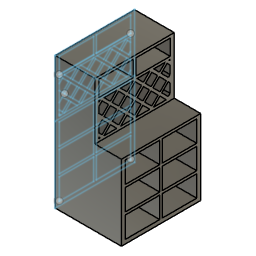
3D Plancha 7 (Autodesk Fusion 360 design; units mm, degrees)
Autodesk Fusion 360 part; units mm, degrees
sketch "Boceto1" plane through (0, 0, 0) normal (1, 0, 0) x (0, 1, 0)
  line L0 (47.0014, 109.9967) -> (107.0014, 109.9967)
  line L1 (107.0014, 109.9967) -> (107.0014, 9.9967)
  line L2 (107.0014, 9.9967) -> (47.0014, 9.9967)
  line L3 (47.0014, 9.9967) -> (47.0014, 109.9967)
  line L4 (47.0014, 66.9967) -> (107.0014, 66.9967)
  line L5 (104.0014, 13.7115) -> (104.0014, 13.2245)
  line L6 (50.0014, 13.2245) -> (50.0014, 13.7115)
  line L7 (76.0014, 64.9967) -> (76.0014, 48.9967)
  line L8 (78.0014, 64.9967) -> (78.0014, 48.9967)
  line L9 (50.0014, 48.9967) -> (76.0014, 48.9967)
  line L10 (78.0014, 48.9967) -> (104.0014, 48.9967)
  line L11 (50.0014, 64.9967) -> (76.0014, 64.9967)
  line L12 (78.0014, 64.9967) -> (104.0014, 64.9967)
  line L13 (76.0014, 46.9967) -> (76.0014, 30.9967)
  line L14 (78.0014, 46.9967) -> (78.0014, 30.9967)
  line L15 (76.0014, 28.9967) -> (76.0014, 12.9967)
  line L16 (78.0014, 28.9967) -> (78.0014, 12.9967)
  line L17 (50.0014, 30.9967) -> (76.0014, 30.9967)
  line L18 (78.0014, 30.9967) -> (104.0014, 30.9967)
  line L19 (50.0014, 12.9967) -> (76.0014, 12.9967)
  line L20 (78.0014, 12.9967) -> (104.0014, 12.9967)
  line L21 (50.0014, 46.9967) -> (76.0014, 46.9967)
  line L22 (78.0014, 46.9967) -> (104.0014, 46.9967)
  line L23 (104.0014, 64.9967) -> (104.0014, 48.9967)
  line L24 (50.0014, 28.9967) -> (76.0014, 28.9967)
  line L25 (78.0014, 28.9967) -> (104.0014, 28.9967)
  line L26 (104.0014, 46.9967) -> (104.0014, 30.9967)
  line L27 (104.0014, 28.9967) -> (104.0014, 12.9967)
  line L28 (50.0014, 12.9967) -> (50.0014, 28.9967)
  line L29 (50.0014, 30.9967) -> (50.0014, 46.9967)
  line L30 (50.0014, 48.9967) -> (50.0014, 64.9967)
  line L31 (103.8321, 93.9967) -> (103.8321, 68.9967)
  line L32 (103.8321, 68.9967) -> (50.0014, 68.9967)
  line L33 (50.0014, 68.9967) -> (50.0014, 93.9967)
  line L34 (104.0014, 107.9967) -> (104.0014, 95.9967)
  line L35 (49.9832, 95.9967) -> (49.9832, 107.9967)
  line L36 (50.0014, 93.9967) -> (103.8321, 93.9967)
  line L37 (76.0014, 95.9967) -> (76.0014, 107.9967)
  line L38 (78.0014, 95.9967) -> (78.0014, 107.9967)
  line L39 (50.0014, 95.9967) -> (76.0014, 95.9967)
  line L40 (78.0014, 95.9967) -> (104.0014, 95.9967)
  line L41 (49.9832, 107.9967) -> (76.0014, 107.9967)
  line L42 (78.0014, 107.9967) -> (104.0014, 107.9967)
  line L43 (104.0014, 95.9967) -> (78.0014, 95.9967)
  line L44 (76.0014, 95.9967) -> (49.9832, 95.9967)
  line L45 (51.0014, 68.9967) -> (50.0014, 69.9967)
  line L46 (50.0014, 72.8251) -> (52.4156, 70.4109)
  line L47 (51.0014, 93.9967) -> (50.0014, 92.9967)
  line L48 (50.0014, 77.666) -> (52.4177, 80.0823)
  line L49 (57.2524, 75.2476) -> (52.4156, 70.4109)
  line L50 (63.5033, 68.9967) -> (58.6666, 73.8334)
  line L51 (57.2524, 75.2476) -> (52.4177, 80.0823)
  line L52 (53.9177, 81.5823) -> (58.7524, 76.7476)
  line L53 (60.1666, 75.3334) -> (65.0033, 70.4967)
  line L54 (53.8298, 68.9967) -> (58.6666, 73.8334)
  line L55 (56.2505, 88.7476) -> (52.4177, 92.5804)
  line L56 (53.8298, 93.9967) -> (58.6667, 89.1598)
  line L57 (58.6667, 89.1598) -> (63.5037, 93.9967)
  line L58 (50.0014, 90.1641) -> (52.4177, 92.5804)
  line L59 (53.8319, 93.9946) -> (53.834, 93.9967)
  line L60 (57.2525, 87.7456) -> (52.5035, 82.9965)
  line L61 (56.2505, 88.7476) -> (57.2525, 87.7456)
  line L62 (50.0014, 85.4986) -> (52.5035, 82.9965)
  line L63 (53.9177, 81.5823) -> (54, 81.5)
  line L64 (53.9177, 81.5823) -> (58.6667, 86.3314)
  line L65 (63.5014, 81.4967) -> (58.7524, 76.7476)
  line L66 (60.1666, 75.3334) -> (64.9156, 80.0825)
  line L67 (63.5014, 81.4967) -> (58.6667, 86.3314)
  line L68 (60.081, 87.7456) -> (64.9156, 82.9109)
  line L69 (101.5872, 92.5825) -> (103.8321, 90.3376)
  line L70 (103.0014, 93.9967) -> (103.8321, 93.166)
  line L71 (102.4156, 70.4109) -> (103.8321, 71.8273)
  line L72 (76.0014, 68.9967) -> (71.2524, 73.7457)
  line L73 (69.7524, 75.2457) -> (64.9156, 80.0825)
  line L74 (60.081, 87.7456) -> (64.9179, 92.5825)
  line L75 (76.0014, 93.9967) -> (71.1667, 89.162)
  line L76 (69.7525, 87.7478) -> (64.9156, 82.9109)
  line L77 (64.9179, 92.5825) -> (69.7525, 87.7478)
  line L78 (66.3321, 93.9967) -> (71.1667, 89.162)
  line L79 (83.6666, 89.16) -> (88.5033, 93.9967)
  line L80 (85.1666, 87.66) -> (90.0033, 92.4967)
  line L81 (77.4156, 92.5825) -> (82.2524, 87.7457)
  line L82 (72.581, 87.7478) -> (77.4177, 82.9111)
  line L83 (77.4177, 82.9111) -> (82.2524, 87.7457)
  line L84 (66.3298, 81.4967) -> (71.1667, 86.3336)
  line L85 (72.581, 87.7478) -> (77.4156, 92.5825)
  line L86 (65.0033, 70.4967) -> (69.7524, 75.2457)
  line L87 (71.1666, 76.66) -> (76.0035, 81.4969)
  line L88 (66.5033, 68.9967) -> (71.2524, 73.7457)
  line L89 (71.1667, 86.3336) -> (76.0035, 81.4969)
  line L90 (66.3298, 81.4967) -> (71.1666, 76.66)
  line L91 (72.6666, 75.16) -> (77.0014, 70.8251)
  line L92 (78.8298, 93.9967) -> (83.6666, 89.16)
  line L93 (100.173, 93.9967) -> (95.8083, 89.632)
  line L94 (91.5033, 93.9967) -> (95.8083, 89.632)
  line L95 (97.2127, 88.208) -> (102.523, 82.824)
  line L96 (90.0033, 92.4967) -> (94.3381, 88.1618)
  line L97 (85.1666, 87.66) -> (89.5014, 83.3251)
  line L98 (97.2127, 88.208) -> (101.5872, 92.5825)
  line L99 (94.3381, 88.1618) -> (89.5014, 83.3251)
  line L100 (90.9156, 81.9109) -> (95.7524, 86.7476)
  line L101 (89.9276, 70.4011) -> (94.7956, 75.2025)
  line L102 (91.3321, 68.9967) -> (96.1667, 73.8314)
  line L103 (97.581, 75.2456) -> (102.4177, 80.0823)
  line L104 (95.7524, 86.7476) -> (101.0897, 81.4103)
  line L105 (102.4177, 80.0823) -> (103.8321, 78.6679)
  line L106 (96.2196, 76.6069) -> (101.0897, 81.4103)
  line L107 (102.523, 82.824) -> (103.8321, 84.1151)
  line L108 (96.1667, 73.8314) -> (101.0014, 68.9967)
  line L109 (90.9156, 81.9109) -> (96.2196, 76.6069)
  line L110 (97.581, 75.2456) -> (102.4156, 70.4109)
  line L111 (78.0014, 68.9967) -> (83.2525, 74.2478)
  line L112 (84.6667, 75.662) -> (89.5014, 80.4967)
  line L113 (88.0872, 81.9109) -> (83.2525, 77.0762)
  line L114 (81.8383, 75.662) -> (77.0014, 70.8251)
  line L115 (72.6666, 75.16) -> (77.5035, 79.9969)
  line L116 (78.9177, 81.4111) -> (83.7524, 86.2457)
  line L117 (78.9177, 81.4111) -> (83.2525, 77.0762)
  line L118 (84.6667, 75.662) -> (89.9276, 70.4011)
  line L119 (77.5035, 79.9969) -> (81.8383, 75.662)
  line L120 (83.2525, 74.2478) -> (88.5037, 68.9967)
  line L121 (83.7524, 86.2457) -> (88.0872, 81.9109)
  line L122 (89.5014, 80.4967) -> (94.7956, 75.2025)
  dimension "d58" = 16
  dimension "d109" = 2
  dimension "d111" = 2
  dimension "d113" = 2
  dimension "d114" = 2
  dimension "d115" = 3
  dimension "d116" = 2
  constraint horizontal L0
  constraint vertical L1
  constraint horizontal L2
  constraint vertical L3
  constraint coincident L3 L4.start
  constraint coincident L1 L4.end
  constraint perpendicular L1 L4
  constraint horizontal L11
  constraint vertical L23
  constraint vertical L28
  constraint coincident L9.start L28
  constraint perpendicular L9 L23
  constraint coincident L17.start L28
  constraint coincident L18.end L23
  constraint perpendicular L17 L23
  constraint vertical L5
  constraint vertical L6
  constraint coincident L5.end L23
  constraint coincident L6.end L28
  constraint coincident L20.end L23
  constraint perpendicular L19 L23
  constraint perpendicular L7 L9
  constraint coincident L8.start L11
  constraint coincident L8.end L9
  constraint perpendicular L8 L9
  constraint collinear L9 L10
  constraint collinear L11 L12
  constraint perpendicular L13 L17
  constraint coincident L14.end L17
  constraint perpendicular L14 L17
  constraint perpendicular L15 L19
  constraint coincident L16.end L19
  constraint perpendicular L16 L19
  constraint collinear L17 L18
  constraint collinear L19 L20
  constraint coincident L21.start L28
  constraint coincident L22.end L23
  constraint perpendicular L21 L23
  constraint coincident L25.end L23
  constraint perpendicular L23 L24
  constraint collinear L21 L22
  constraint collinear L23 L26
  constraint coincident L16.start L24
  constraint collinear L24 L25
  constraint collinear L26 L27
  constraint collinear L28 L29
  constraint collinear L29 L30
  constraint horizontal L39
  constraint vertical L31
  constraint horizontal L32
  constraint vertical L33
  constraint horizontal L41
  constraint vertical L34
  constraint horizontal L43
  constraint vertical L35
  constraint perpendicular L31 L36
  constraint coincident L38.start L39
  constraint coincident L38.end L41
  constraint collinear L39 L40
  constraint collinear L41 L42
  constraint collinear L43 L44
  constraint coincident L32 L45.start
  constraint coincident L32 L54.start
  constraint coincident L36 L92.start
  constraint coincident L32 L72.start
  constraint coincident L36 L47.start
  constraint coincident L36 L56.start
  constraint coincident L32 L111.start
  constraint coincident L36 L70.start
  constraint coincident L36 L93.start
  constraint coincident L33 L45.end
  constraint perpendicular L45 L75
  constraint coincident L33 L46.start
  constraint perpendicular L46 L54
  constraint coincident L33 L47.end
  constraint coincident L33 L58.start
  constraint coincident L36 L59.end
  constraint coincident L36 L57.end
  constraint coincident L33 L48.start
  constraint coincident L33 L62.start
  constraint coincident L32 L88.start
  constraint perpendicular L54 L62
  constraint coincident L32 L50.start
  constraint coincident L52.start L62
  constraint collinear L48 L64
  constraint collinear L52 L62
  constraint coincident L49.start L50
  constraint collinear L49 L75
  constraint collinear L50 L51
  constraint coincident L53.start L54
  constraint collinear L52 L53
  constraint collinear L54 L66
  constraint collinear L55 L72
  constraint coincident L68.start L64
  constraint collinear L56 L68
  constraint coincident L56 L59.start
  constraint collinear L58 L59
  constraint perpendicular L60 L62
  constraint perpendicular L60 L61
  constraint collinear L62 L63
  constraint collinear L64 L74
  constraint coincident L65.start L72
  constraint collinear L65 L75
  constraint coincident L84.start L68
  constraint collinear L66 L84
  constraint collinear L67 L72
  constraint collinear L68 L90
  constraint coincident L32 L120.end
  constraint perpendicular L77 L111
  constraint coincident L36 L79.end
  constraint coincident L78.start L74
  constraint coincident L36 L78.start
  constraint coincident L32 L102.start
  constraint perpendicular L78 L93
  constraint coincident L36 L94.start
  constraint perpendicular L77 L88
  constraint coincident L32 L108.end
  constraint perpendicular L81 L93
  constraint coincident L31 L105.end
  constraint perpendicular L88 L96
  constraint coincident L31 L69.end
  constraint perpendicular L69 L93
  constraint coincident L31 L70.end
  constraint perpendicular L70 L111
  constraint coincident L31 L107.end
  constraint perpendicular L94 L101
  constraint coincident L31 L71.end
  constraint perpendicular L71 L92
  constraint collinear L72 L73
  constraint collinear L75 L76
  constraint collinear L77 L89
  constraint coincident L82.start L84
  constraint collinear L78 L82
  constraint collinear L79 L86
  constraint coincident L116.end L81
  constraint coincident L80.start L92
  constraint collinear L80 L88
  constraint collinear L81 L121
  constraint coincident L82.end L86
  constraint coincident L116.start L88
  constraint collinear L82 L117
  constraint collinear L83 L86
  constraint collinear L84 L85
  constraint collinear L86 L87
  constraint coincident L91.start L90
  constraint collinear L88 L115
  constraint collinear L89 L119
  constraint collinear L90 L91
  constraint collinear L92 L97
  constraint collinear L93 L99
  constraint coincident L69.start L111
  constraint coincident L95.start L111
  constraint collinear L94 L95
  constraint collinear L96 L104
  constraint coincident L100.start L111
  constraint collinear L97 L109
  constraint collinear L98 L111
  constraint collinear L99 L113
  constraint coincident L112.end L121
  constraint collinear L100 L111
  constraint collinear L101 L106
  constraint coincident L102.end L121
  constraint coincident L103.start L109
  constraint collinear L102 L103
  constraint collinear L104 L105
  constraint collinear L106 L107
  constraint collinear L108 L121
  constraint collinear L109 L110
  constraint coincident L111.end L119
  constraint coincident L112.start L117
  constraint collinear L111 L112
  constraint collinear L113 L114
  constraint collinear L115 L116
  constraint collinear L117 L118
  constraint collinear L119 L120
  constraint collinear L121 L122
  constraint coincident L36 L75.start
  measures "d58" distance of L7.start L7.end
  measures "d109" distance of L36 L40
  measures "d111" distance of L4 L12
  measures "d113" distance of L10 L22
  measures "d114" distance of L18 L25
  measures "d115" distance of L2 L20
  measures "d116" distance of L4 L32
sketch "Boceto2" plane through (0, 0, 0) normal (1, 0, 0) x (0, 1, 0)
sketch "Boceto3" plane through (0, 0, 0) normal (1, 0, 0) x (0, 1, 0)
extrude "Extruir1" add sketch "Boceto1" along normal blind 50 contours L1 L2 L3 L4
extrude "Extruir2" add sketch "Boceto1" along normal blind 30 contours L0 L1 L3 L4 | L31 L32 L33 L36 L45 L46 L47 L48 L49 L50 L51 L54 L55 L56 L57 L58 L60 L61 L62 L69 L70 L71 L72 L75 L78 L79 L88 L92 L93 L94 L95 L98 L102 L103 L105 L107 L108 L110 L111 L120
